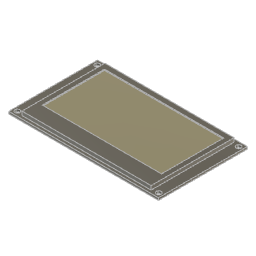
UHF-ROTARIES (Autodesk Fusion 360 archive; units mm, degrees)
design "SD1309 LCD Panel"
Autodesk Fusion 360 part; units mm, degrees
sketch "Sketch1" plane through (0, 0, 0) normal (0, 0, 1) x (1, 0, 0)
  line L0 (36.125, -21.42) -> (-36.125, -21.42)
  line L1 (-36.125, -21.42) -> (-36.125, 21.42)
  line L2 (-36.125, 21.42) -> (36.125, 21.42)
  line L3 (36.125, 21.42) -> (36.125, -21.42)
  line L4 (36.125, -21.42) -> (-36.125, 21.42) construction
  line L5 (-36.125, -21.42) -> (36.125, 21.42) construction
  line L6 (31.15, -20) -> (-31.15, -20)
  line L7 (-31.15, -20) -> (-31.15, 20)
  line L8 (-31.15, 20) -> (31.15, 20)
  line L9 (31.15, 20) -> (31.15, -20)
  line L10 (31.15, -20) -> (-31.15, 20) construction
  line L11 (-31.15, -20) -> (31.15, 20) construction
  line L12 (28.75, -15) -> (-28.75, 15) construction
  line L13 (-28.75, -15) -> (28.75, 15) construction
  line L14 (36.125, -18.0538) -> (34.125, -18.0538) construction
  line L15 (34.125, -21.42) -> (34.125, 22) construction
  line L16 (-36.125, 20.5191) -> (-34.125, 20.5191) construction
  line L17 (-34.125, 20.5191) -> (-34.125, -21.42) construction
  circle A0 centre (-34.125, -19.236) radius 1.2
  line L18 (-34.125, -21.42) -> (-34.125, -20.67)
  line L19 (-34.1139, 21.42) -> (-34.1139, 19.27) construction
  circle A1 centre (-34.1139, 19.27) radius 1.2
  line L20 (34.125, 21.42) -> (34.125, 19.27) construction
  circle A2 centre (34.125, 19.27) radius 1.2
  line L21 (34.125, -21.42) -> (34.125, -19.27) construction
  circle A3 centre (34.125, -19.27) radius 1.2
  line L22 (0, 21.42) -> (0, 17.42) construction
  line L23 (0, 17.42) -> (28.75, 17.42) construction
  line L24 (28.75, 17.42) -> (-28.75, 17.42)
  line L25 (-28.75, 17.42) -> (-28.75, -12.58)
  line L26 (-28.75, -12.58) -> (28.75, -12.58)
  line L27 (28.75, -12.58) -> (28.75, 17.42)
  circle A4 centre (34.125, 19.27) radius 2
  circle A5 centre (-34.1139, 19.27) radius 2
  circle A6 centre (-34.125, -19.236) radius 2
  circle A7 centre (34.125, -19.27) radius 2
  line L28 (38.125, 23.42) -> (-38.125, 23.42)
  line L29 (-38.125, 23.42) -> (-38.125, -23.42)
  line L30 (-38.125, -23.42) -> (38.125, -23.42)
  line L31 (38.125, -23.42) -> (38.125, 23.42)
  line L32 (38.125, 23.42) -> (-38.125, -23.42) construction
  line L33 (-38.125, 23.42) -> (38.125, -23.42) construction
  line L34 (37.25, 22.25) -> (-37.25, 22.25)
  line L35 (-37.25, 22.25) -> (-37.25, -22.25)
  line L36 (-37.25, -22.25) -> (37.25, -22.25)
  line L37 (37.25, -22.25) -> (37.25, 22.25)
  line L38 (37.25, 22.25) -> (-37.25, -22.25) construction
  line L39 (-37.25, 22.25) -> (37.25, -22.25) construction
  dimension "d1" = 72.25
  dimension "d2" = 42.84
  dimension "d3" = 62.3
  dimension "d4" = 40
  dimension "d5" = 57.5
  dimension "d6" = 30
  dimension "d7" = 2
  dimension "d8" = 2
  dimension "d9" = 2.4
  dimension "d11" = 0.75
  dimension "d12" = 2.15
  dimension "d13" = 2.4
  dimension "d14" = 2.4
  dimension "d15" = 2.15
  dimension "d16" = 2.4
  dimension "d17" = 2.15
  dimension "d18" = 2.4
  dimension "d19" = 4
  dimension "d20" = 28.75
  dimension "d21" = 57.5
  dimension "d22" = 30
  dimension "d24" = 30
  dimension "d27" = 30
  dimension "d28" = 4
  dimension "d29" = 4
  dimension "d30" = 4
  dimension "d31" = 4
  dimension "d37" = 76.25
  dimension "d38" = 46.84
  dimension "d39" = 74.5
  dimension "d40" = 44.5
  constraint horizontal L0
  constraint perpendicular L0 L1
  constraint parallel L0 L2
  constraint parallel L1 L3
  constraint coincident L4 origin
  constraint coincident L5 origin
  constraint horizontal L6
  constraint perpendicular L6 L7
  constraint parallel L6 L8
  constraint parallel L7 L9
  constraint coincident L10 origin
  constraint coincident L11 origin
  constraint coincident L12 origin
  constraint coincident L13 origin
  constraint coincident L3 L14.start
  constraint perpendicular L3 L14
  constraint coincident L0 L15.start
  constraint perpendicular L2 L15
  constraint coincident L1 L16.start
  constraint perpendicular L1 L16
  constraint coincident L0 L17.end
  constraint perpendicular L0 L17
  constraint coincident L17 A0.centre
  constraint perpendicular L0 L18
  constraint coincident L2 L19.start
  constraint perpendicular L16 L19
  constraint coincident L19.end A1.centre
  constraint coincident L2 L20.start
  constraint coincident L15 L20.start
  constraint perpendicular L2 L20
  constraint coincident L20.end A2.centre
  constraint perpendicular L0 L21
  constraint coincident L21.end A3.centre
  constraint midpoint L2 L22.start
  constraint perpendicular L8 L22
  constraint perpendicular L22 L23
  constraint horizontal L24
  constraint vertical L25
  constraint horizontal L26
  constraint vertical L27
  constraint concentric A2 A4
  constraint concentric A1 A5
  constraint concentric A0 A6
  constraint concentric A3 A7
  constraint horizontal L28
  constraint perpendicular L28 L29
  constraint parallel L28 L30
  constraint parallel L29 L31
  constraint coincident L32 origin
  constraint coincident L33 origin
  constraint horizontal L34
  constraint perpendicular L34 L35
  constraint parallel L34 L36
  constraint parallel L35 L37
  constraint coincident L38 origin
  constraint coincident L39 origin
  measures "d1" distance of L1.end L2.end
  measures "d2" distance of L0.end L1.end
  measures "d3" distance of L7.end L8.end
  measures "d4" distance of L6.end L7.end
  measures "d5" distance of L12.end L13.end
  measures "d6" distance of L13.start L12.end
  measures "d7" distance of L14.start L14.end
  measures "d8" distance of L16.start L16.end
  measures "d9" diameter of A0
  measures "d11" distance of L17.end L18.end
  measures "d12" distance of L19.start L19.end
  measures "d13" diameter of A1
  measures "d14" diameter of A1
  measures "d15" distance of L20.start L20.end
  measures "d16" diameter of A2
  measures "d17" distance of L15.start L21.end
  measures "d18" diameter of A3
  measures "d19" distance of L22.start L22.end
  measures "d20" distance of L22.end L23.end
  measures "d21" distance of L23.end L24.end
  measures "d22" distance of L23.end L26.end
  measures "d24" distance of L24.end L25.end
  measures "d27" distance of L23.end L26.end
  measures "d28" diameter of A4
  measures "d29" diameter of A5
  measures "d30" diameter of A6
  measures "d31" diameter of A7
  measures "d37" distance of L29.end L30.end
  measures "d38" distance of L28.end L29.end
  measures "d39" distance of L35.end L36.end
  measures "d40" distance of L34.end L35.end
extrude "Extrude1" add sketch "Sketch1" against normal blind 3.1 contours A7 | A4 | A6 | A5 makes body 1 at (36.1225, 19.1703, -2.0667) makes body 2 at (36.1225, -19.3697, -2.0667) makes body 3 at (-32.1164, 19.1703, -2.0667) makes body 4 at (-32.1349, -19.0369, -1.0333)
extrude "Extrude2" add sketch "Sketch1" along normal blind 1 contours A7 | A4 | L0 L1 L2 L3 L18 A6 | L0 L1 L18 A6 | A6 | L6 L7 L8 L9 | A0 | A1 | A2 | A3 | A5 | L28 L29 L30 L31 | L34 L35 L36 L37 bodies 1 2 3 4
extrude "Extrude3" add sketch "Sketch1" against normal blind 3 contours L34 L35 L36 L37 bodies 1
fillet "Fillet1" radius 1 4 edges at (-38.125, 0, 1) (0, -23.42, 1) (38.125, 0, 1) (0, 23.42, 1) on bodies 1
chamfer "Chamfer1" distance 3 distance2 0.9 4 edges at (28.75, 2.42, 1) (0, 17.42, 1) (-28.75, 2.42, 1) (0, -12.58, 1) measured on face at (9.5833, -19.1401, 1) measured on face at (9.5833, -19.1401, 1) measured on face at (9.5833, -19.1401, 1) measured on face at (9.5833, -19.1401, 1) on bodies 1
sketch "Sketch2" plane through (0, 0, -3.1) normal (0, 0, -1) x (1, 0, 0)
  circle A0 centre (-34.125, 19.236) radius 1.2
  circle A1 centre (-34.125, 19.236) radius 2
  line L0 (-36.1253, 21.4221) -> (36.1242, 21.4221)
  line L1 (36.1242, 21.4221) -> (36.1242, -21.4189)
  line L2 (36.1242, -21.4189) -> (-36.1253, -21.4189)
  line L3 (-36.1253, -21.4189) -> (-36.1253, 21.4221)
  line L4 (-31.15, -20) -> (31.15, -20)
  line L5 (31.15, -20) -> (31.15, 20)
  line L6 (31.15, 20) -> (-31.15, 20)
  line L7 (-31.15, 20) -> (-31.15, -20)
  circle A2 centre (34.1232, 19.2725) radius 1.2039
  circle A3 centre (-34.125, 19.236) radius 1.2
  circle A4 centre (-34.1138, -19.2699) radius 1.1936
  circle A5 centre (34.1249, -19.2699) radius 1.194
  line L8 (-28.7509, 12.58) -> (28.75, 12.58)
  line L9 (28.75, 12.58) -> (28.75, -17.42)
  line L10 (28.75, -17.42) -> (-28.7509, -17.42)
  line L11 (-28.7509, -17.42) -> (-28.7509, 12.58)
  constraint horizontal L0
  constraint vertical L1
  constraint horizontal L2
  constraint vertical L3
  constraint horizontal L4
  constraint vertical L5
  constraint horizontal L6
  constraint vertical L7
  constraint concentric A0 A3
  constraint horizontal L8
  constraint vertical L9
  constraint horizontal L10
  constraint vertical L11
extrude "Extrude1'" add sketch "Sketch2" against normal blind 1.12 separate body contours L0 L1 L2 L3 | L4 L5 L6 L7 | L8 L9 L10 L11 makes body 5 in component "Component"
extrude "Extrude2'" add sketch "Sketch2" against normal blind 3 contours L4 L5 L6 L7 bodies 5 in component "Component"
extrude "Extrude3'" add sketch "Sketch2" against normal blind 2.5 contours L8 L9 L10 L11 bodies 5 in component "Component"
extrude "Extrude4" add sketch "Sketch2" against normal blind 1.12 contours A1 bodies 5 in component "Component"
component "Component" placed x (1, 0, 0) y (0, 1, 0) z (0, 0, 1) at (0, 0, 0)
hidden bodies 1
equation "d20 = ( 57.5 / 2 ) * 1 mm"
named bodies: "SD1309 Frame", "SD1309 Panel"
